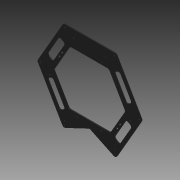
# Autodesk Inventor part: Bottom Plate
Saved by Autodesk Inventor 2015 (Build 190159000, 159)
## iProperties
Created: 2016-10-01
Part Number: Bottom Plate
Material: PVC, Unplasticized
Document SubType Name: Modeling
Designer: James Yelland
Density: 1.29 g/cm^3
Appearance: Smooth - White
Mass: 31.7822 g
Surface Area: 281.879 cm^2
Volume: 24.6374 cm^3
Author: James Yelland
Autodesk Inventor part; units mm, degrees
ref_plane "YZ Plane" through (0, 0, 0) normal (1, 0, 0) x (0, 1, 0)
ref_plane "XZ Plane" through (0, 0, 0) normal (0, 1, 0) x (-1, 0, 0)
ref_plane "XY Plane" through (0, 0, 0) normal (0, 0, 1) x (1, 0, 0)
sketch "Sketch1" plane through (0, 0, 0) normal (0, 1, 0) x (-1, 0, 0)
  line L0 (72.6878, -41.9663) -> (62.1878, -60.1529)
  line L1 (72.6878, -41.9663) -> (83.1878, -23.7798)
  line L2 (81.7237, -18.3157) -> (77.3936, -15.8157)
  line L3 (71.9295, -17.2797) -> (50.9295, -53.6529)
  line L4 (52.3936, -59.117) -> (56.7237, -61.617)
  arc A0 (56.7237, -61.617) -> (62.1878, -60.1529) centre (58.7237, -58.1529) ccw
  arc A1 (50.9295, -53.6529) -> (52.3936, -59.117) centre (54.3936, -55.6529) ccw
  arc A2 (77.3936, -15.8157) -> (71.9295, -17.2797) centre (75.3936, -19.2798) ccw
  arc A3 (83.1878, -23.7798) -> (81.7237, -18.3157) centre (79.7237, -21.7798) ccw
  line L5 (55.5994, -35.5644) -> (57.3314, -36.5644)
  line L6 (57.3314, -36.5644) -> (54.8314, -40.8945)
  line L7 (53.0994, -39.8945) -> (55.5994, -35.5644)
  line L8 (54.8314, -40.8945) -> (53.0994, -39.8945)
  line L9 (61.0994, -26.0381) -> (58.5994, -30.3683)
  line L10 (60.3314, -31.3683) -> (62.8314, -27.0381)
  line L11 (58.5994, -30.3683) -> (60.3314, -31.3683)
  line L12 (62.8314, -27.0381) -> (61.0994, -26.0381)
  line L13 (-72.6878, -41.9663) -> (-83.1878, -23.7798)
  line L14 (-72.6878, -41.9663) -> (-62.1878, -60.1529)
  line L15 (-56.7237, -61.617) -> (-52.3936, -59.117)
  line L16 (-50.9295, -53.6529) -> (-71.9294, -17.28)
  line L17 (-77.3936, -15.8157) -> (-81.7237, -18.3157)
  arc A4 (-81.7237, -18.3157) -> (-83.1878, -23.7798) centre (-79.7237, -21.7798) ccw
  arc A5 (-71.9294, -17.28) -> (-77.3936, -15.8157) centre (-75.3936, -19.2798) ccw
  arc A6 (-52.3936, -59.117) -> (-50.9295, -53.6529) centre (-54.3936, -55.6529) ccw
  arc A7 (-62.1878, -60.1529) -> (-56.7237, -61.617) centre (-58.7237, -58.1529) ccw
  line L18 (-58.5994, -30.3683) -> (-60.3314, -31.3683)
  line L19 (-61.0994, -26.0381) -> (-58.5994, -30.3683)
  line L20 (-62.8314, -27.0381) -> (-61.0994, -26.0381)
  line L21 (-60.3314, -31.3683) -> (-62.8314, -27.0381)
  line L22 (-54.8314, -40.8945) -> (-53.0994, -39.8945)
  line L23 (-53.0994, -39.8945) -> (-55.5994, -35.5644)
  line L24 (-55.5994, -35.5644) -> (-57.3314, -36.5644)
  line L25 (-57.3314, -36.5644) -> (-54.8314, -40.8945)
  line L26 (103.5566, -2.5) -> (54.8095, -86.9325)
  line L27 (-54.8095, -86.9325) -> (-103.5566, -2.5)
  line L28 (-103.5566, 2.5) -> (-53.9434, 88.4327)
  line L29 (-49.6132, 90.9327) -> (49.6132, 90.9327)
  line L30 (53.9434, 88.4327) -> (103.5566, 2.5)
  line L31 (2.1497, -66.9563) -> (48.3297, -88.9468)
  line L32 (-2.1497, -66.9563) -> (-48.3297, -88.9468)
  arc A8 (48.3297, -88.9468) -> (54.8095, -86.9325) centre (50.4794, -84.4325) ccw
  arc A9 (2.1497, -66.9563) -> (-2.1497, -66.9563) centre (0, -71.4706) ccw
  arc A10 (-54.8095, -86.9325) -> (-48.3297, -88.9468) centre (-50.4794, -84.4325) ccw
  arc A11 (-103.5566, 2.5) -> (-103.5566, -2.5) centre (-99.2265, 0) ccw
  arc A12 (-49.6132, 90.9327) -> (-53.9434, 88.4327) centre (-49.6132, 85.9327) ccw
  arc A13 (53.9434, 88.4327) -> (49.6132, 90.9327) centre (49.6132, 85.9327) ccw
  arc A14 (103.5566, -2.5) -> (103.5566, 2.5) centre (99.2265, 0) ccw
  circle A15 centre (49.6132, 85.9327) radius 1.6
  circle A16 centre (-49.6132, 85.9327) radius 1.6
  circle A17 centre (-99.2265, 0) radius 1.6
  circle A18 centre (99.2265, 0) radius 1.6
  line L33 (0, -52.117) -> (-38.9295, -52.117)
  line L34 (0, -52.117) -> (38.9295, -52.117)
  line L35 (66.4295, -9.4856) -> (43.2596, -49.617)
  line L36 (-43.2596, -49.617) -> (-66.4295, -9.4856)
  arc A19 (38.9295, -52.117) -> (43.2596, -49.617) centre (38.9295, -47.117) ccw
  arc A20 (-43.2596, -49.617) -> (-38.9295, -52.117) centre (-38.9295, -47.117) ccw
  circle A21 centre (-25, 62.282) radius 1.6
  circle A22 centre (25, 62.282) radius 1.6
  circle A23 centre (24, -57.282) radius 1.6
  circle A24 centre (-24, -57.282) radius 1.6
  line L37 (49.6132, 90.9327) -> (32.6132, 90.9327)
  line L38 (-49.6132, 90.9327) -> (-32.6132, 90.9327)
  line L39 (66.4295, -9.4856) -> (68.9295, -5.1554)
  line L40 (-66.4295, -9.4856) -> (-68.9295, -5.1554)
  circle A25 centre (80.7596, -11.9856) radius 1.6
  circle A26 centre (-80.7596, -11.9856) radius 1.6
  line L41 (72.6878, 41.9663) -> (62.1878, 60.1529)
  line L42 (72.6878, 41.9663) -> (83.1878, 23.7798)
  line L43 (81.7237, 18.3157) -> (77.3936, 15.8157)
  line L44 (71.9295, 17.2797) -> (50.9295, 53.6529)
  line L45 (52.3936, 59.117) -> (56.7237, 61.617)
  arc A27 (62.1878, 60.1529) -> (56.7237, 61.617) centre (58.7237, 58.1529) ccw
  arc A28 (52.3936, 59.117) -> (50.9295, 53.6529) centre (54.3936, 55.6529) ccw
  arc A29 (71.9295, 17.2797) -> (77.3936, 15.8157) centre (75.3936, 19.2798) ccw
  arc A30 (81.7237, 18.3157) -> (83.1878, 23.7798) centre (79.7237, 21.7798) ccw
  line L46 (55.5994, 35.5644) -> (57.3314, 36.5644)
  line L47 (53.0994, 39.8945) -> (55.5994, 35.5644)
  line L48 (54.8314, 40.8945) -> (53.0994, 39.8945)
  line L49 (57.3314, 36.5644) -> (54.8314, 40.8945)
  line L50 (62.8314, 27.0381) -> (61.0994, 26.0381)
  line L51 (61.0994, 26.0381) -> (58.5994, 30.3683)
  line L52 (58.5994, 30.3683) -> (60.3314, 31.3683)
  line L53 (60.3314, 31.3683) -> (62.8314, 27.0381)
  arc A31 (-56.7237, 61.617) -> (-62.1878, 60.1529) centre (-58.7237, 58.1529) ccw
  line L54 (-56.7237, 61.617) -> (-52.3936, 59.117)
  arc A32 (-50.9295, 53.6529) -> (-52.3936, 59.117) centre (-54.3936, 55.6529) ccw
  line L55 (-72.6878, 41.9663) -> (-62.1878, 60.1529)
  line L56 (-54.8314, 40.8945) -> (-53.0994, 39.8945)
  line L57 (-57.3314, 36.5644) -> (-54.8314, 40.8945)
  line L58 (-53.0994, 39.8945) -> (-55.5994, 35.5644)
  line L59 (-55.5994, 35.5644) -> (-57.3314, 36.5644)
  line L60 (-58.5994, 30.3683) -> (-60.3314, 31.3683)
  line L61 (-60.3314, 31.3683) -> (-62.8314, 27.0381)
  line L62 (-61.0994, 26.0381) -> (-58.5994, 30.3683)
  line L63 (-50.9295, 53.6529) -> (-71.9294, 17.28)
  line L64 (-72.6878, 41.9663) -> (-83.1878, 23.7798)
  line L65 (-62.8314, 27.0381) -> (-61.0994, 26.0381)
  arc A33 (-83.1878, 23.7798) -> (-81.7237, 18.3157) centre (-79.7237, 21.7798) ccw
  line L66 (-77.3936, 15.8157) -> (-81.7237, 18.3157)
  arc A34 (-77.3936, 15.8157) -> (-71.9294, 17.28) centre (-75.3936, 19.2798) ccw
  line L67 (66.4295, 9.4856) -> (43.2596, 49.617)
  line L68 (-43.2596, 49.617) -> (-66.4295, 9.4856)
  line L69 (66.4295, 9.4856) -> (70.4626, 2.5)
  line L70 (-66.4295, 9.4856) -> (-68.9295, 5.1554)
  line L71 (43.2596, 49.617) -> (40.2831, 54.7724)
  line L72 (-43.2596, 49.617) -> (-40.2831, 54.7724)
  line L73 (-35.953, 57.2724) -> (35.953, 57.2724)
  line L74 (68.9295, -5.1554) -> (70.4626, -2.5)
  line L75 (-68.9295, -5.1554) -> (-70.4626, -2.5)
  line L76 (-70.4626, 2.5) -> (-68.9295, 5.1554)
  arc A35 (40.2831, 54.7724) -> (35.953, 57.2724) centre (35.953, 52.2724) ccw
  arc A36 (-35.953, 57.2724) -> (-40.2831, 54.7724) centre (-35.953, 52.2724) ccw
  arc A37 (-70.4626, 2.5) -> (-70.4626, -2.5) centre (-66.1325, 0) ccw
  arc A38 (70.4626, -2.5) -> (70.4626, 2.5) centre (66.1325, 0) ccw
  circle A39 centre (80.7596, -11.9856) radius 1.6
  circle A40 centre (-80.7596, -11.9856) radius 1.6
  circle A41 centre (-32.6132, 75.9327) radius 1.6
  circle A42 centre (32.6132, 75.9327) radius 1.6
  line L77 (-80.7596, -11.9856) -> (-77.7596, -11.9856) construction
  circle A43 centre (50.4794, -84.4325) radius 1.45
  circle A44 centre (50.4794, -76.4325) radius 1.45
  circle A45 centre (-50.4794, -76.4325) radius 1.45
  circle A46 centre (-50.4794, -84.4325) radius 1.45
  point P0 (60.1878, -63.617)
  point P1 (85.1878, -20.3157)
  point P2 (73.9295, -13.8157)
  point P3 (48.9295, -57.117)
  point P4 (-85.1878, -20.3157)
  point P5 (-60.1878, -63.617)
  point P6 (-48.9295, -57.117)
  point P7 (-73.9295, -13.8157)
  point P8 (105, 0)
  point P9 (52.5, -90.9327)
  point P10 (-105, 0)
  point P11 (-52.5, 90.9327)
  point P12 (52.5, 90.9327)
  point P13 (-86.25, -15.1554)
  point P14 (-88.75, -10.8253)
  point P15 (61.9338, 57.2724)
  point P16 (71.4295, -0.8253)
  point P17 (-71.4295, -0.8253)
  point P18 (60.1878, 63.617)
  point P19 (85.1878, 20.3157)
  point P20 (73.9295, 13.8157)
  point P21 (48.9295, 57.117)
  point P22 (-48.9295, 57.117)
  point P23 (-60.1878, 63.617)
  point P24 (-73.9295, 13.8157)
  point P25 (-85.1878, 20.3157)
  point P26 (-88.75, 10.8253)
  point P27 (-86.25, 15.1554)
  point P28 (71.4295, 0.8253)
  dimension "d11" = 360
  dimension "d30" = 360
  dimension "d90" = 360
  dimension "d72" = 5
  dimension "d83" = 3.2
  dimension "d84" = 3.2
  dimension "d85" = 3.2
  dimension "d86" = 3.2
  dimension "d92" = 17
  dimension "d95" = 17
  dimension "d100" = 10
  dimension "d102" = 10
  dimension "d107" = 3.2
  dimension "d110" = 3.2
  dimension "d111" = 5
  dimension "d112" = 3.2
  constraints: 156 end point, 58 point on circle, 47 centre point, 46 point on line, 8 coincident, 8 tangent, 3 equal radius, 1 horizontal, 1 parallel
  measures "d72" radius of A19
  measures "d83" diameter of A21
  measures "d84" diameter of A22
  measures "d85" diameter of A23
  measures "d86" diameter of A24
  measures "d92" distance of L29.end L37.end
  measures "d95" distance of L29.start L38.end
  measures "d100" distance of L35.start point (71.429, -0.825)
  measures "d102" distance of L36.end point (-71.429, -0.825)
  measures "d107" diameter of A25
  measures "d110" diameter of A26
  measures "d111" radius of A35
  measures "d112" diameter of A40
extrude "Extrusion1" add sketch "Sketch1" along normal blind 2
body "Solid1"
